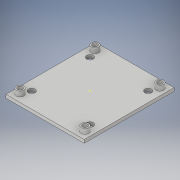
# Autodesk Inventor part: Box1_Buttom
Saved by Autodesk Inventor 2017 (Build 210142000, 142)
## iProperties
Created: 2017-11-12
Part Number: Box1_Buttom
Material: Generic
Document SubType Name: Modeling
Designer: Arthur Bondar
Density: 1 g/cm^3
Appearance: Default
Author: Arthur Bondar
Autodesk Inventor part; units mm, degrees
ref_plane "YZ Plane" through (0, 0, 0) normal (1, 0, 0) x (0, 1, 0)
ref_plane "XZ Plane" through (0, 0, 0) normal (0, 1, 0) x (-1, 0, 0)
ref_plane "XY Plane" through (0, 0, 0) normal (0, 0, 1) x (1, 0, 0)
sketch "Sketch1" plane through (0, 0, 0) normal (0, 1, 0) x (-1, 0, 0)
  point P0 (0, 0)
sketch "Sketch2" plane through (0, 0, 0) normal (0, 1, 0) x (-1, 0, 0)
  line L0 (23.5, 27) -> (-23.5, 27)
  line L1 (-23.5, 27) -> (-23.5, -27)
  line L2 (-23.5, -27) -> (23.5, -27)
  line L3 (23.5, -27) -> (23.5, 27)
  dimension "d4" = 47
  dimension "d5" = 54
  constraints: 8 end point, 2 parallel, 1 horizontal, 1 perpendicular
  measures "d4" distance of L2.end L1.end
  measures "d5" distance of L1.end L0.end
extrude "Extrusion1" add sketch "Sketch2" along normal blind 2
sketch "Sketch3" plane through (0, 2, 0) normal (0, 1, 0) x (1, 0, 0)
  point P0 (0, 0)
sketch "Sketch4" plane through (0, 2, 0) normal (0, 1, 0) x (1, 0, 0)
  circle A0 centre (19.5, 22.5) radius 1.5
  circle A1 centre (19.5, -22.5) radius 1.5
  circle A2 centre (-19.5, -22.5) radius 1.5
  circle A3 centre (-19.5, 22.5) radius 1.5
  circle A4 centre (-19.5, 22.5) radius 2.25
  circle A5 centre (19.5, 22.5) radius 2.25
  circle A6 centre (19.5, -22.5) radius 2.25
  circle A7 centre (-19.5, -22.5) radius 2.25
  dimension "d24" = 3
  dimension "d27" = 3
  dimension "d30" = 3
  dimension "d33" = 3
  dimension "d34" = 4.5
  dimension "d35" = 4.5
  dimension "d36" = 4.5
  dimension "d37" = 4.5
  constraints: 8 centre point, 4 coincident
  measures "d24" diameter of A0
  measures "d27" diameter of A1
  measures "d30" diameter of A2
  measures "d33" diameter of A3
  measures "d34" diameter of A4
  measures "d35" diameter of A5
  measures "d36" diameter of A6
  measures "d37" diameter of A7
extrude "Extrusion2" add sketch "Sketch4" along normal blind 3
sketch "Sketch5" plane through (0, 2, 0) normal (0, 1, 0) x (1, 0, 0)
  circle A0 centre (-17.5, -17.5) radius 2
  circle A1 centre (-17.5, 17.5) radius 2
  circle A2 centre (17.5, 17.5) radius 2
  circle A3 centre (17.5, -17.5) radius 2
  dimension "d42" = 4
  dimension "d43" = 4
  dimension "d44" = 4
  dimension "d45" = 4
  constraints: 4 centre point
  measures "d42" diameter of A0
  measures "d43" diameter of A1
  measures "d44" diameter of A2
  measures "d45" diameter of A3
extrude "Extrusion3" cut sketch "Sketch5" against normal through all
body "Solid1"
